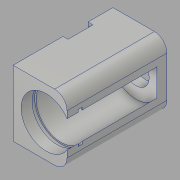
# Autodesk Inventor part: linear bearing mount
Saved by Autodesk Inventor 2017 (Build 210142000, 142)
## iProperties
Created: 2016-12-06
Part Number: linear bearing mount
Material: Aluminum 6061
Document SubType Name: Modeling
Designer: qupec
Density: 2.7 g/cm^3
Appearance: Aluminum - Flat
Mass: 2.94313 g
Surface Area: 9.3484 cm^2
Volume: 1.09005 cm^3
Author: qupec
Autodesk Inventor part; units mm, degrees
ref_plane "YZ Plane" through (0, 0, 0) normal (1, 0, 0) x (0, 1, 0)
sketch "Sketch1" plane through (0, 0, 0) normal (0, 0, 1) x (1, 0, 0)
  circle A0 centre (0, 0) radius 6.35
  line L0 (8.382, -8.382) -> (-8.382, -8.382)
  line L1 (-8.382, -8.382) -> (-8.382, 8.382)
  line L2 (-8.382, 8.382) -> (8.382, 8.382)
  line L3 (8.382, 8.382) -> (8.382, -8.382)
  dimension "d10" = 12.7
  dimension "d11" = 2.032
  dimension "d26" = 16.764
  dimension "d28" = 0
  dimension "d29" = 8.382
  dimension "d37" = 2.032
  dimension "d38" = 2.032
  dimension "d39" = 2.032
  constraints: 8 end point, 2 parallel, 1 centre point, 1 horizontal, 1 perpendicular
  measures "d10" diameter of A0
  measures "d11" distance edge to line of A0 L3
  measures "d26" distance of L1.end L2.end
  measures "d28" distance of point (0, 0) A0.centre
  measures "d29" distance from line of A0.centre L1
  measures "d37" distance edge to line of A0 L0
  measures "d38" distance edge to line of A0 L2
  measures "d39" distance edge to line of A0 L1
extrude "Extrusion2" add sketch "Sketch1" along normal blind 25.4
sketch "Sketch2" plane through (-8.382, -8.382, 0) normal (-1, 0, 0) x (0, 0, 1)
  line L0 (25.4, 14.732) -> (25.4, 2.032) projected
  line L1 (0, 2.032) -> (0, 14.732) projected
  line L2 (0, 14.732) -> (25.4, 14.732) projected
  line L3 (0, 2.032) -> (25.4, 2.032) projected
  line L4 (0, 0) -> (0, 16.764) projected
  line L5 (0, 0) -> (25.4, 0) projected
  line L6 (25.4, 16.764) -> (25.4, 0) projected
  line L7 (0, 16.764) -> (25.4, 16.764) projected
  circle A0 centre (6.35, 15.748) radius 1.4224
  circle A1 centre (6.35, 1.016) radius 1.4224
  point P0 (0, 8.382)
  dimension "d17" = 2.032
  dimension "d18" = 2.8448
  dimension "d19" = 2.8448
  dimension "d20" = 1.016
  dimension "d21" = 1.016
  dimension "d22" = 6.35
  dimension "d23" = 6.35
  constraints: 2 centre point
  measures "d17" distance between parallel lines of L2 L7
  measures "d18" diameter of A0
  measures "d19" diameter of A1
  measures "d20" distance from line of A0.centre L7
  measures "d21" distance from line of L5 A1.centre
  measures "d22" distance from line of L4 A0.centre
  measures "d23" distance from line of L4 A1.centre
extrude "Extrusion3" [suppressed]
sketch "Sketch3" plane through (0, 0, 0) normal (0, 0, -1) x (-1, 0, 0)
  circle A0 centre (0, 0) radius 3.3655
  circle A1 centre (0, 0) radius 6.35 projected
  dimension "d30" = 6.731
  constraints: 1 centre point, 1 coincident
  measures "d30" diameter of A0
extrude "Extrusion4" add sketch "Sketch3" against normal blind 2.54
ref_plane "Work Plane1" through (0, 0, 21.59) normal (0, 0, 1) x (1, 0, 0)
sketch "Sketch4" plane through (0, 0, 21.59) normal (0, 0, 1) x (1, 0, 0)
  circle A0 centre (0, 0) radius 6.35 projected
  circle A1 centre (0, 0) radius 6.7056
  dimension "d34" = 0.3556
  constraints: 1 centre point, 1 coincident
  measures "d34" radial gap between concentric circles of A0 A1
extrude "Extrusion5" cut sketch "Sketch4" along normal blind 1.016
sketch "Sketch5" plane through (-8.382, -8.382, 0) normal (-1, 0, 0) x (0, 0, 1)
  line L0 (0, 0) -> (0, 16.764) projected
  line L1 (0, 0) -> (25.4, 0) projected
  line L2 (25.4, 16.764) -> (25.4, 0) projected
  line L3 (0, 16.764) -> (25.4, 16.764) projected
  line L4 (25.4, 14.732) -> (25.4, 2.032) projected
  line L5 (21.59, 2.032) -> (21.59, 14.732) projected
  line L6 (2.54, 14.732) -> (2.54, 2.032) projected
  line L7 (0, 16.764) -> (25.4, 16.764) projected
  line L8 (6.35, 0) -> (12.7, 0)
  line L9 (12.7, 0) -> (12.7, 16.764)
  line L10 (12.7, 16.764) -> (6.35, 16.764)
  line L11 (6.35, 16.764) -> (6.35, 0)
  point P0 (0, 8.382)
  dimension "d40" = 6.35
  dimension "d41" = 6.35
  constraints: 8 end point, 2 parallel, 1 horizontal, 1 midpoint, 1 perpendicular, 1 point on line
  measures "d40" distance between parallel lines of L11 L9
  measures "d41" distance between parallel lines of L0 L11
ref_plane "Work Plane2" through (-6.35, 0, 0) normal (-1, 0, 0) x (0, -1, 0)
extrude "Extrusion6" cut sketch "Sketch5" against normal blind 1.27 contours L11 L3 L9 L1
sketch "Sketch7" plane through (0, 0, 0) normal (0, 0, -1) x (-1, 0, 0)
  line L0 (7.112, -8.382) -> (7.112, 8.382) projected
  line L1 (7.112, 8.382) -> (7.112, -8.382) projected
  point P0 (0, 0)
  dimension "d46" = 7.112
  measures "d46" distance from line of L0 point (0, 0)
sketch "Sketch8" plane through (0, 0, 25.4) normal (0, 0, 1) x (1, 0, 0)
  circle A0 centre (0, 0) radius 6.35 projected
  circle A1 centre (0, 0) radius 6.7056 projected
  circle A2 centre (0, 0) radius 6.7056 projected
  line L0 (8.382, -8.382) -> (-8.382, -8.382) projected
  line L1 (-8.382, 8.382) -> (8.382, 8.382) projected
  line L2 (8.382, 8.382) -> (8.382, -8.382) projected
  line L3 (5.334, 8.382) -> (8.382, 8.382)
  line L4 (8.382, 8.382) -> (8.382, -8.382)
  line L5 (8.382, -8.382) -> (5.334, -8.382)
  line L6 (5.334, -8.382) -> (5.334, 8.382)
  point P0 (5.207, -8.382)
  point P1 (5.207, -8.382)
  point P2 (-5.207, -8.382)
  dimension "d50" = 3.048
  constraints: 8 end point, 2 parallel, 2 point on line, 1 horizontal, 1 perpendicular
  measures "d50" distance between parallel lines of L2 L6
extrude "Extrusion8" cut sketch "Sketch8" against normal through all contours A0 L6 | A0 L6 A1 | L6 L1 L2 L0 A1 picked at (5.5198, -0.7897) picked at (6.4961, 0.8835)
fillet "Fillet3" radius 3.175 2 edges at (5.334, -8.382, 12.7) (5.334, 8.382, 12.7)
equation "\"d37\" = d11"
equation "\"d38\" = d11"
equation "\"d39\" = d11"
equation "\"d20\" = 0.5 * d17"
equation "\"d21\" = d20"
equation "\"d23\" = d22"
body "Solid2"
